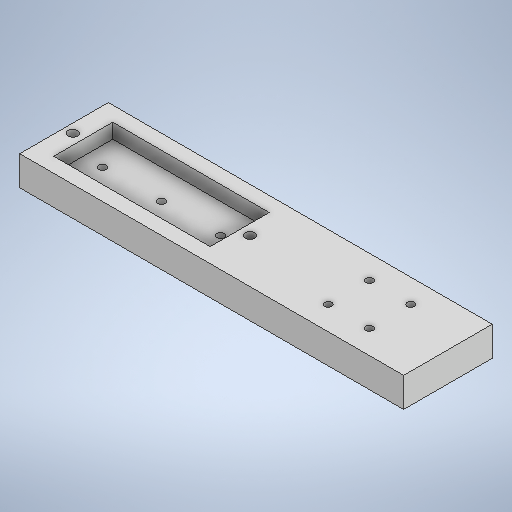
# Autodesk Inventor part: prortezione penna correnti parassite
Saved by Autodesk Inventor 2025.2 (Build 292293000, 293)
## iProperties
Created: 2025-04-29
Part Number: prortezione penna correnti parassite
Material: Generico
Document SubType Name: Modeling
Designer: caset
Density: 1 g/cm^3
Appearance: Default
Author: caset
Autodesk Inventor part; units mm, degrees
ref_plane "YZ Plane" through (0, 0, 0) normal (1, 0, 0) x (0, 1, 0)
ref_plane "XZ Plane" through (0, 0, 0) normal (0, 1, 0) x (-1, 0, 0)
ref_plane "XY Plane" through (0, 0, 0) normal (0, 0, 1) x (1, 0, 0)
sketch "Schizzo1" plane through (0, 0, 0) normal (0, 1, 0) x (-1, 0, 0)
  line L0 (0, 0) -> (130, 0)
  line L1 (130, 0) -> (130, -30)
  line L2 (130, -30) -> (0, -30)
  line L3 (0, -30) -> (0, 0)
  dimension "d0" = 30
  dimension "d1" = 130
  constraints: 8 end point, 2 parallel, 1 horizontal, 1 perpendicular
  measures "d0" distance of L2.end L0.start
  measures "d1" distance of L0.start L0.end
extrude "Estrusione1" add sketch "Schizzo1" along normal blind 10
sketch "Schizzo2" plane through (0, 10, 0) normal (0, 1, 0) x (1, 0, 0)
  line L0 (-185.4023, 5) -> (-60, 5)
  line L1 (-60, 5) -> (-60, 25)
  line L2 (-60, 25) -> (-185.4023, 25)
  line L3 (-185.4023, 25) -> (-185.4023, 5)
  line L4 (-130, 0) -> (0, 0) projected
  line L5 (-130, 30) -> (-130, 0) projected
  point P0 (-130, 25)
  point P1 (-130, 5)
  dimension "d4" = 20
  dimension "d5" = 5
  dimension "d6" = 70
  constraints: 8 end point, 2 parallel, 1 horizontal, 1 perpendicular
  measures "d4" distance of L0.end L1.end
  measures "d5" distance between parallel lines of L4 L0
  measures "d6" distance between parallel lines of L1 L5
extrude "Estrusione2" cut sketch "Schizzo2" against normal blind 5 contours L5 L2 L1 L0
sketch "Schizzo3" plane through (0, 5, 0) normal (0, 1, 0) x (1, 0, 0)
  circle A0 centre (-127, 15) radius 1.65
  circle A1 centre (-117, 15) radius 1.3
  circle A2 centre (-97, 15) radius 1.3
  circle A3 centre (-77, 15) radius 1.3
  circle A4 centre (-67, 15) radius 1.65
  line L0 (-130, 0) -> (0, 0) projected
  line L1 (-130, 5) -> (-130, 25) projected
  line L2 (-145.516, 5) -> (-124, 5)
  line L3 (-124, 5) -> (-124, 25)
  line L4 (-124, 25) -> (-145.516, 25)
  line L5 (-145.516, 25) -> (-145.516, 5)
  line L6 (-60, 5) -> (-130, 5) projected
  line L7 (-70, 5) -> (-43.6658, 5)
  line L8 (-43.6658, 5) -> (-43.6658, 25)
  line L9 (-43.6658, 25) -> (-70, 25)
  line L10 (-70, 25) -> (-70, 5)
  dimension "d9" = 3.3
  dimension "d10" = 2.6
  dimension "d11" = 2.6
  dimension "d12" = 2.6
  dimension "d13" = 3.3
  dimension "d14" = 15
  dimension "d15" = 63
  dimension "d16" = 60
  dimension "d18" = 10
  dimension "d19" = 0
  dimension "d20" = 0
  dimension "d21" = 0
  dimension "d22" = 40
  dimension "d23" = 20
  dimension "d39" = 6
  dimension "d40" = 0
  dimension "d41" = 20
  dimension "d42" = 0
  dimension "d43" = 20
  dimension "d44" = 54
  constraints: 16 end point, 5 centre point, 4 parallel, 2 horizontal, 2 perpendicular
  measures "d9" diameter of A0
  measures "d10" diameter of A1
  measures "d11" diameter of A2
  measures "d12" diameter of A3
  measures "d13" diameter of A4
  measures "d14" distance from line of A4.centre L0
  measures "d15" distance from line of A4.centre L1
  measures "d16" distance of A0.centre A4.centre
  measures "d18" distance of A1.centre A0.centre
  measures "d19" vertical distance of A0.centre A1.centre
  measures "d20" vertical distance of A1.centre A2.centre
  measures "d21" vertical distance of A2.centre A3.centre
  measures "d22" distance of A3.centre A1.centre
  measures "d23" distance of A2.centre A3.centre
  measures "d39" distance between parallel lines of L3 L1
  measures "d40" distance between parallel lines of L6 L2
  measures "d41" distance of L4.end L2.start
  measures "d42" distance between parallel lines of L7 L6
  measures "d43" distance of L7.end L8.end
  measures "d44" distance between parallel lines of L3 L10
extrude "Estrusione3" cut sketch "Schizzo3" along normal through all both and the other way through all contours A0 | A1 | A2 | A3 | A4
sketch "Schizzo4" plane through (0, 10, 0) normal (0, 1, 0) x (1, 0, 0)
  circle A0 centre (-33.5752, 8) radius 1.25
  circle A1 centre (-19.5752, 8) radius 1.25
  circle A2 centre (-19.5752, 22) radius 1.25
  circle A3 centre (-33.5752, 22) radius 1.25
  line L0 (-130, 0) -> (0, 0) projected
  dimension "d26" = 14
  dimension "d27" = 14
  dimension "d28" = 14
  dimension "d29" = 14
  dimension "d30" = 0
  dimension "d31" = 0
  dimension "d32" = 8
  dimension "d33" = 2.5
  dimension "d34" = 2.5
  dimension "d35" = 2.5
  dimension "d36" = 2.5
  constraints: 4 centre point
  measures "d26" distance of A3.centre A0.centre
  measures "d27" distance of A0.centre A1.centre
  measures "d28" distance of A2.centre A1.centre
  measures "d29" distance of A3.centre A2.centre
  measures "d30" horizontal distance of A0.centre A3.centre
  measures "d31" vertical distance of A3.centre A2.centre
  measures "d32" distance from line of A0.centre L0
  measures "d33" diameter of A0
  measures "d34" diameter of A3
  measures "d35" diameter of A2
  measures "d36" diameter of A1
extrude "Estrusione4" cut sketch "Schizzo4" against normal through all
sketch "Schizzo5" plane through (0, 5, 0) normal (0, 1, 0) x (1, 0, 0)
  line L0 (-60, 5) -> (-130, 5) projected
  line L1 (-130, 25) -> (-60, 25) projected
  line L2 (-60, 5) -> (-70.5, 5)
  line L3 (-70.5, 5) -> (-70.5, 25)
  line L4 (-70.5, 25) -> (-60, 25)
  line L5 (-60, 25) -> (-60, 5)
  line L6 (-130, 30) -> (-130, 0) projected
  line L7 (-130, 5) -> (-123.5, 5)
  line L8 (-123.5, 5) -> (-123.5, 25)
  line L9 (-123.5, 25) -> (-130, 25)
  line L10 (-130, 25) -> (-130, 5)
  point P0 (0, 0)
  point P1 (-123.5, 5)
  point P2 (-123.5, 25)
  dimension "d45" = 6.5
  dimension "d46" = 53
  constraints: 16 end point, 4 parallel, 4 point on line, 2 horizontal, 2 perpendicular
  measures "d45" distance between parallel lines of L8 L6
  measures "d46" distance between parallel lines of L3 L8
extrude "Estrusione5" add sketch "Schizzo5" along normal blind 5 contours L0 L3 L1 L5 | L0 L6 L1 L8
sketch "Schizzo6" plane through (0, 0, 0) normal (0, -1, 0) x (1, 0, 0)
  circle A0 centre (-127, -15) radius 1.65 projected
  circle A1 centre (-127, -15) radius 1.65
  circle A2 centre (-67, -15) radius 1.65 projected
  circle A3 centre (-67, -15) radius 1.65
  point P0 (0, 0)
  dimension "d49" = 3.3
  dimension "d50" = 3.3
  constraints: 2 centre point, 2 coincident
  measures "d49" diameter of A1
  measures "d50" diameter of A3
extrude "Estrusione6" cut sketch "Schizzo6" against normal blind 50
